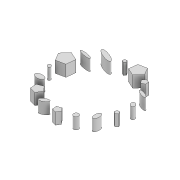
# Autodesk Inventor part: simple_ring1
Saved by Autodesk Inventor 2021 (Build 250183000, 183)
## iProperties
Created: 2022-04-11
Part Number: simple_ring1
Material: Generic
Document SubType Name: Modeling
Designer: Derm
Density: 1 g/cm^3
Appearance: Default
Author: Derm
Autodesk Inventor part; units mm, degrees
ref_plane "YZ Plane" through (0, 0, 0) normal (1, 0, 0) x (0, 1, 0)
ref_plane "XZ Plane" through (0, 0, 0) normal (0, 1, 0) x (-1, 0, 0)
ref_plane "XY Plane" through (0, 0, 0) normal (0, 0, 1) x (1, 0, 0)
sketch "Sketch1" plane through (0, 0, 0) normal (0, 1, 0) x (-1, 0, 0)
  circle A0 centre (0, 0) radius 10000 construction
  circle A1 centre (0, 0) radius 10000 construction
  circle A2 centre (0, 0) radius 10000 construction
  circle A3 centre (0, 0) radius 10000 construction
  circle A4 centre (0, 0) radius 10000 construction
  circle A5 centre (0, 0) radius 10000 construction
  circle A6 centre (0, 0) radius 10000 construction
  circle A7 centre (0, 0) radius 10000 construction
  circle A8 centre (0, 0) radius 10000 construction
  circle A9 centre (0, 0) radius 10000 construction
  circle A10 centre (0, 0) radius 10000 construction
  circle A11 centre (0, 0) radius 10000 construction
  circle A12 centre (0, 0) radius 10000 construction
  circle A13 centre (0, 0) radius 10000 construction
  circle A14 centre (0, 0) radius 10000 construction
  circle A15 centre (0, 0) radius 10000 construction
  ellipse E0 centre (9941.0978, 1083.7777) end of major axis (10285.5807, 665.9604) minor radius 397.3786
  ellipse E1 centre (4805.5735, -8769.633) end of major axis (2883.6714, -7980.3132) minor radius 611.4415
  ellipse E2 centre (2803.0134, 9599.1206) end of major axis (3821.0865, 10171.2822) minor radius 510.0188
  ellipse E3 centre (-8769.633, -4805.5735) end of major axis (-7550.2878, -5306.3552) minor radius 399.5638
  ellipse E4 centre (-4805.5735, 8769.633) end of major axis (-5050.8301, 8172.4618) minor radius 637.4066
  ellipse E5 centre (-7795.7643, 6263.0711) end of major axis (-7213.0774, 6263.0711) minor radius 1130.3941
  ellipse E6 centre (8769.633, 4805.5735) end of major axis (7544.8504, 4805.5735) minor radius 723.4556
  ellipse E7 centre (7795.7643, -6263.0711) end of major axis (9375.2429, -6550.32) minor radius 376.7629
  line L0 (5919.3647, 6442.8953) -> (4870.2052, 7704.589)
  line L1 (4870.2052, 7704.589) -> (5745.939, 9092.2838)
  line L2 (5745.939, 9092.2838) -> (7336.3318, 8688.2326)
  line L3 (7336.3318, 8688.2326) -> (7443.5148, 7050.8205)
  line L4 (7443.5148, 7050.8205) -> (5919.3647, 6442.8953)
  line L5 (8090.2446, -1454.2488) -> (10415.6036, -951.1959)
  line L6 (10415.6036, -951.1959) -> (11612.6108, -3007.2918)
  line L7 (11612.6108, -3007.2918) -> (10027.0429, -4781.0819)
  line L8 (10027.0429, -4781.0819) -> (7850.1009, -3821.2485)
  line L9 (7850.1009, -3821.2485) -> (8090.2446, -1454.2488)
  line L10 (-1183.8363, -8681.432) -> (-1429.8865, -10855.4681)
  line L11 (-1429.8865, -10855.4681) -> (-3573.5514, -11293.2746)
  line L12 (-3573.5514, -11293.2746) -> (-4652.359, -9389.8178)
  line L13 (-4652.359, -9389.8178) -> (-3175.4338, -7775.6103)
  line L14 (-3175.4338, -7775.6103) -> (-1183.8363, -8681.432)
  line L15 (600.7452, -9918.1823) -> (956.3064, -9474.6253)
  line L16 (956.3064, -9474.6253) -> (1488.0286, -9675.7174)
  line L17 (1488.0286, -9675.7174) -> (1461.0899, -10243.5562)
  line L18 (1461.0899, -10243.5562) -> (912.7186, -10393.4078)
  line L19 (912.7186, -10393.4078) -> (600.7452, -9918.1823)
  line L20 (-5457.0462, -7767.6634) -> (-5987.2702, -8553.6559)
  line L21 (-5987.2702, -8553.6559) -> (-6898.6417, -8292.2679)
  line L22 (-6898.6417, -8292.2679) -> (-6931.6762, -7344.7288)
  line L23 (-6931.6762, -7344.7288) -> (-6040.7212, -7020.5054)
  line L24 (-6040.7212, -7020.5054) -> (-5457.0462, -7767.6634)
  line L25 (-9896.0177, 2303.6638) -> (-10165.7765, 2931.0719)
  line L26 (-10165.7765, 2931.0719) -> (-9652.436, 3381.5074)
  line L27 (-9652.436, 3381.5074) -> (-9065.4154, 3032.4839)
  line L28 (-9065.4154, 3032.4839) -> (-9215.9572, 2366.3399)
  line L29 (-9215.9572, 2366.3399) -> (-9896.0177, 2303.6638)
  line L30 (-333.9797, 10542.1263) -> (-280.4653, 9413.7255)
  line L31 (-280.4653, 9413.7255) -> (-1337.1014, 9014.1353)
  line L32 (-1337.1014, 9014.1353) -> (-2043.6528, 9895.5758)
  line L33 (-2043.6528, 9895.5758) -> (-1423.6895, 10839.9261)
  line L34 (-1423.6895, 10839.9261) -> (-333.9797, 10542.1263)
  ellipse E8 centre (-9941.0978, -1083.7777) end of major axis (-9512.2663, -1668.1835) minor radius 541.7232
  point P0 (6263.0711, 7795.7643)
  point P1 (-1083.7777, 9941.0978)
  point P2 (-9599.1206, 2803.0134)
  point P3 (-6263.0711, -7795.7643)
  point P4 (-2803.0134, -9599.1206)
  point P5 (1083.7777, -9941.0978)
  point P6 (9599.1206, -2803.0134)
  point P7 (6263.0711, 7795.7643)
  point P8 (9599.1206, -2803.0134)
  point P9 (-2803.0134, -9599.1206)
  point P10 (1083.7777, -9941.0978)
  point P11 (-6263.0711, -7795.7643)
  point P12 (-9599.1206, 2803.0134)
  point P13 (-1083.7777, 9941.0978)
  dimension "d0" = 20000
  dimension "d3" = 360
  constraints: 70 end point, 19 coincident, 6 centre point, 182 other
extrude "Extrusion1" add sketch "Sketch1" along normal mid plane 3000
body "Solid1"
